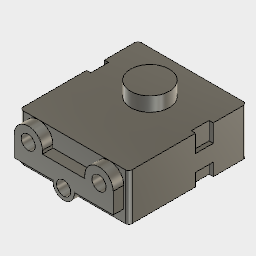
1092 Tactile On Off Switch (Autodesk Fusion 360 design; units mm, degrees)
Autodesk Fusion 360 part; units mm, degrees
note: some values were not read from the file. Set by a fixed rule: which sketch regions a step uses.
sketch "main body" plane through (0, 0, 0) normal (0, 0, 1) x (1, 0, 0)
  line L0 (7.7, -8.35) -> (-7.7, -8.35)
  line L1 (-7.7, -8.35) -> (-7.7, 8.35)
  line L2 (-7.7, 8.35) -> (7.7, 8.35)
  line L3 (7.7, 8.35) -> (7.7, -8.35)
  line L4 (7.7, -8.35) -> (-7.7, 8.35) construction
  line L5 (-7.7, -8.35) -> (7.7, 8.35) construction
  dimension "d1" = 15.4
  dimension "d2" = 16.7
  measures "d1" distance of L1.end L2.end
  measures "d2" distance of L0.end L1.end
extrude "Extrude1" add sketch "main body" along normal blind 6.6
sketch "top actuator" plane through (0, 0, 6.6) normal (0, 0, 1) x (-1, 0, 0)
  line L0 (-7.7, -8.35) -> (7.7, -8.35)
  line L1 (7.7, -8.35) -> (7.7, 8.35)
  line L2 (7.7, 8.35) -> (-7.7, 8.35)
  line L3 (-7.7, 8.35) -> (-7.7, -8.35)
  circle A0 centre (0, -2.35) radius 2.725
  dimension "d5" = 5.45
  dimension "d6" = 6
  measures "d5" diameter of A0
  measures "d6" distance of L0 A0.centre
extrude "Extrude2" add sketch "top actuator" along normal blind 2 contours A0
fillet "Fillet1" radius 0.5 4 edges at (-7.7, -8.35, 3.3) (7.7, 8.35, 3.3) (7.7, -8.35, 3.3) (-7.7, 8.35, 3.3)
sketch "side cuts" plane through (-7.7, 0, 0) normal (-1, 0, 0) x (0, -1, 0)
  line L0 (-7.85, 6.6) -> (-7.85, 0)
  line L1 (-7.85, 0) -> (7.85, 0)
  line L2 (7.85, 0) -> (7.85, 6.6)
  line L3 (7.85, 6.6) -> (-7.85, 6.6)
  line L4 (-8.35, 0) -> (-8.35, 6.6)
  line L5 (-8.35, 6.6) -> (-8.35, 0)
  line L6 (0.375, 8.6) -> (-5.075, 8.6)
  line L7 (-2.35, 8.6) -> (-2.35, 0) construction
  line L8 (-1.1, 4.1) -> (-3.6, 4.1)
  line L9 (-3.6, 4.1) -> (-3.6, 6.6)
  line L10 (-3.6, 6.6) -> (-1.1, 6.6)
  line L11 (-1.1, 6.6) -> (-1.1, 4.1)
  line L12 (-1.1, 4.1) -> (-3.6, 6.6) construction
  line L13 (-3.6, 4.1) -> (-1.1, 6.6) construction
  line L14 (-1.1, 0) -> (-3.6, 0)
  line L15 (-3.6, 0) -> (-3.6, 1.8)
  line L16 (-3.6, 1.8) -> (-1.1, 1.8)
  line L17 (-1.1, 1.8) -> (-1.1, 0)
  line L18 (-1.1, 0) -> (-3.6, 1.8) construction
  line L19 (-3.6, 0) -> (-1.1, 1.8) construction
  point P0 (-2.35, 5.35)
  point P1 (-2.35, 0.9)
  dimension "d10" = 8.6
  dimension "d11" = 2.5
  dimension "d12" = 2.5
  dimension "d13" = 2.5
  dimension "d14" = 1.8
  measures "d10" distance of L7.start L7.end
  measures "d11" distance of L8.end L9.end
  measures "d12" distance of L9.end L10.end
  measures "d13" distance of L15.end L16.end
  measures "d14" distance of L14.end L15.end
extrude "Extrude3" cut sketch "side cuts" against normal blind 0.6 contours L3 L8 L9 L10 L11 | L1 L14 L15 L16 L17
mirror "Mirror1" about plane through (0, 0, 0) normal (1, 0, 0) of "Extrude3"
sketch "Sketch4" plane through (0, -8.35, 0) normal (0, -1, 0) x (1, 0, 0)
  line L0 (7.2, 0) -> (7.2, 6.6)
  line L1 (7.2, 6.6) -> (-7.2, 6.6)
  line L2 (-7.2, 6.6) -> (-7.2, 0)
  line L3 (-7.2, 0) -> (7.2, 0)
  line L4 (-7.2, 2.9) -> (7.2, 2.9) construction
  circle A0 centre (-5, 4.6) radius 2
  line L5 (0, 6.6) -> (0, 0) construction
  line L6 (-7, 4.6) -> (-3, 4.6)
  line L7 (-3, 4.6) -> (-3, 1.7)
  line L8 (-3, 1.7) -> (-7, 1.7)
  line L9 (-7, 1.7) -> (-7, 4.6)
  line L10 (-3, 1.7) -> (0, 1.7)
  line L11 (0, 1.7) -> (0, 4.15)
  line L12 (0, 4.15) -> (-3, 4.15)
  line L13 (-3, 4.15) -> (-3, 1.7)
  circle A1 centre (-5, 4.6) radius 1
  circle A2 centre (0, 1.5) radius 1
  circle A3 centre (0, 1.5) radius 1.5
  circle A4 centre (5, 4.6) radius 2
  circle A5 centre (5, 4.6) radius 1
  line L14 (7, 1.7) -> (7, 4.6)
  line L15 (3, 1.7) -> (7, 1.7)
  line L16 (3, 4.6) -> (3, 1.7)
  line L17 (0, 4.15) -> (3, 4.15)
  line L18 (3, 1.7) -> (0, 1.7)
  dimension "d18" = 3.7
  dimension "d19" = 4
  dimension "d20" = 5
  dimension "d21" = 1.7
  dimension "d22" = 2
  dimension "d23" = 2.45
  dimension "d24" = 3
  dimension "d25" = 2
  dimension "d26" = 2
  dimension "d27" = 3
  measures "d18" distance of L1 L4
  measures "d19" diameter of A0
  measures "d20" distance of A0.centre L5
  measures "d21" distance of L3 L8
  measures "d22" distance of L1 A0.centre
  measures "d23" distance of L7.end L12.end
  measures "d24" distance of L7.end L10.end
  measures "d25" diameter of A1
  measures "d26" diameter of A2
  measures "d27" diameter of A3
extrude "Extrude4" add sketch "Sketch4" along normal blind 1.5 contours L10 A2 A3 L18 | A4 | L10 L11 A2 A3 | L7 L10 L11 L12 L13 A3 | A0 L6 A1 | A4 L14 L15 L16 | A0 L7 L8 L9 L13 | L11 A2 A3 L18 | L11 A3 L16 L17 L18 | A0 L6 A1
